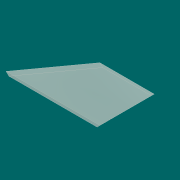
# Autodesk Inventor part: mirror
Saved by Autodesk Inventor 2016 (Build 200138000, 138)
## iProperties
Created: 2015-10-13
Part Number: mirror
Material: Glass
Document SubType Name: Modeling
Designer: Sawaiz
Density: 2.18 g/cm^3
Appearance: Clear
Author: Sawaiz
Autodesk Inventor part; units mm, degrees
ref_plane "XZ Plane" through (0, 0, 0) normal (0, 1, 0) x (-1, 0, 0)
ref_plane "XY Plane" through (0, 0, 0) normal (0, 0, 1) x (1, 0, 0)
sketch "Sketch1" plane through (0, 0, 0) normal (1, 0, 0) x (0, 1, 0)
  line L0 (-50, -50) -> (50, -50)
  line L1 (50, -50) -> (50, 50)
  line L2 (50, 50) -> (-50, 50)
  line L3 (-50, 50) -> (-50, -50)
  line L4 (-50, -50) -> (50, 50) construction
  line L5 (50, -50) -> (-50, 50) construction
  line L6 (-47, -47) -> (47, -47)
  line L7 (47, -47) -> (47, 47)
  line L8 (47, 47) -> (-47, 47)
  line L9 (-47, 47) -> (-47, -47)
  line L10 (-47, -47) -> (47, 47) construction
  line L11 (47, -47) -> (-47, 47) construction
  point P0 (0, 0)
  dimension "d0" = 100
  dimension "d1" = 100
  dimension "d7" = 3
  dimension "d8" = 3
  constraints: 24 end point, 4 midpoint, 4 parallel, 2 horizontal, 2 perpendicular
  measures "d0" distance of L2.end L1.end
  measures "d1" distance of L1.end L0.end
  measures "d7" distance between parallel lines of L2 L8
  measures "d8" distance between parallel lines of L3 L9
ref_plane "Work Plane1" through (-79, 0, 0) normal (1, 0, 0) x (0, 1, 0)
sketch "Sketch2" plane through (-79, 0, 0) normal (1, 0, 0) x (0, 1, 0)
  line L0 (-26, -26) -> (26, -26)
  line L1 (26, -26) -> (26, 26)
  line L2 (26, 26) -> (-26, 26)
  line L3 (-26, 26) -> (-26, -26)
  line L4 (-26, -26) -> (26, 26) construction
  line L5 (26, -26) -> (-26, 26) construction
  line L6 (-29, -29) -> (29, -29)
  line L7 (29, -29) -> (29, 29)
  line L8 (29, 29) -> (-29, 29)
  line L9 (-29, 29) -> (-29, -29)
  line L10 (-29, -29) -> (29, 29) construction
  line L11 (29, -29) -> (-29, 29) construction
  point P0 (0, 0)
  dimension "d4" = 52
  dimension "d5" = 52
  dimension "d9" = 3
  constraints: 24 end point, 4 midpoint, 4 parallel, 2 horizontal, 2 perpendicular, 1 point on line
  measures "d4" distance of L2.end L1.end
  measures "d5" distance of L1.end L0.end
  measures "d9" distance between parallel lines of L8 L2
loft "Loft1" add profiles "Sketch1", "Sketch2" contours L3 L2 L1 L0 | L9 L8 L7 L6 / L3 L2 L1 L0 | L9 L8 L7 L6
sketch "Sketch3" plane through (0, -50, -50) normal (1, 0, 0) x (0, 0, -1)
  line L0 (-3, 3) -> (-97, 3)
  line L1 (-97, 3) -> (-97, 97)
  line L2 (-97, 97) -> (-3, 97)
  line L3 (-3, 97) -> (-3, 3)
  line L4 (-3, 3) -> (-97, 97) construction
  line L5 (-97, 3) -> (-3, 97) construction
  line L6 (0, 100) -> (-100, 100) projected
  line L7 (-100, 100) -> (-100, 0) projected
  point P0 (-50, 50)
  dimension "d14" = 3
  dimension "d15" = 3
  constraints: 12 end point, 2 midpoint, 2 parallel, 1 horizontal, 1 perpendicular
  measures "d14" distance between parallel lines of L6 L2
  measures "d15" distance between parallel lines of L7 L1
sketch "Sketch4" plane through (-79, -29, -29) normal (-1, 0, 0) x (0, 0, 1)
  line L0 (3, 55) -> (55, 55)
  line L1 (55, 55) -> (55, 3)
  line L2 (55, 3) -> (3, 3)
  line L3 (3, 3) -> (3, 55)
  line L4 (3, 55) -> (55, 3) construction
  line L5 (55, 55) -> (3, 3) construction
  line L6 (58, 58) -> (58, 0) projected
  line L7 (58, 0) -> (0, 0) projected
  point P0 (29, 29)
  dimension "d16" = 3
  dimension "d17" = 3
  constraints: 12 end point, 2 midpoint, 2 parallel, 1 horizontal, 1 perpendicular
  measures "d16" distance between parallel lines of L6 L1
  measures "d17" distance between parallel lines of L7 L2
loft "Loft2" cut profiles "Sketch4", "Sketch3"
sketch "Sketch5" plane through (0, 0, 0) normal (1, 0, 0) x (0, 1, 0)
  line L0 (50, 50) -> (-50, 50) projected
  line L1 (-50, 50) -> (-50, -50) projected
  line L2 (-50, -50) -> (50, -50) projected
  line L3 (50, -50) -> (50, 50) projected
  line L4 (0, 0) -> (-50, 50)
  line L5 (0, 0) -> (50, 50)
  line L6 (26, 26) -> (47, 47) projected
  constraints: 4 end point, 1 collinear
extrude "Extrusion1" cut sketch "Sketch5" against normal through all contours L3 L2 L1 L4 L5
equation "\"d0\" = width"
equation "\"d1\" = height"
equation "\"d7\" = mirrorThickness"
equation "\"d8\" = mirrorThickness"
equation "\"d4\" = detectorWidth"
equation "\"d5\" = detectorHeight"
equation "\"d9\" = mirrorThickness"
equation "\"d14\" = mirrorThickness"
equation "\"d15\" = mirrorThickness"
equation "\"d16\" = mirrorThickness"
equation "\"d17\" = mirrorThickness"
equation "\"acrylicThickness\" = 6.35"
equation "\"height\" = 100"
equation "\"width\" = 100"
equation "\"mirrorAngle\" = 5deg"
equation "\"detectorWidth\" = 52"
equation "\"detectorHeight\" = 52"
equation "\"mirrorThickness\" = 3"
equation "\"d3\" = fresnelThickness - depth + aerogelThickness"
equation "\"fresnelThickness\" = 0.1"
equation "\"focalLength\" = 76.2"
equation "\"ior\" = 1.49"
equation "\"fresnelAngle\" = 90deg"
equation "\"centerThickness\" = 1.524"
equation "\"fresnelEffectiveDiameter\" = 76.2"
equation "\"depth\" = 100"
equation "\"aerogelThickness\" = 20"
body "Solid1"
